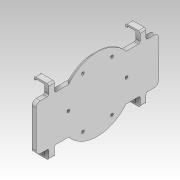
# Autodesk Inventor part: PhoneHOldER
Saved by Autodesk Inventor 2020 (Build 240168000, 168)
## iProperties
Created: 2022-08-28
Part Number: PhoneHOldER
Material: Generic
Document SubType Name: Modeling
Designer: DDeGo
Density: 1 g/cm^3
Appearance: Default
Author: DDeGo
Autodesk Inventor part; units mm, degrees
ref_plane "YZ Plane" through (0, 0, 0) normal (1, 0, 0) x (0, 1, 0)
ref_plane "XZ Plane" through (0, 0, 0) normal (0, 1, 0) x (-1, 0, 0)
sketch "Sketch1" plane through (0, 0, 0) normal (0, 0, 1) x (1, 0, 0)
  line L0 (0, 0) -> (0, 44)
  line L1 (-5, 0) -> (0, 0)
  line L2 (0, 44) -> (-1, 44)
  line L3 (-1, 44) -> (-5, 40)
  line L4 (-5, 40) -> (-5, 0)
  dimension "d0" = 44
  dimension "d3" = 1
  dimension "d19" = 5
  dimension "d20" = 45
  constraints: 10 end point, 2 horizontal, 1 perpendicular, 1 vertical
  measures "d0" distance of L0.start L0.end
  measures "d3" distance of L0.end L2.end
  measures "d19" distance between parallel lines of L0 L4
  measures "d20" angle of L0 L3
revolve "Revolution1" add sketch "Sketch1" angle 360 about axis through (-5, 0, 0) along (1, 0, 0)
sketch "Sketch2" plane through (0, 0, 0) normal (1, 0, 0) x (0, 0, -1)
  line L0 (0, 0) -> (35, 0) construction
  circle A0 centre (35, 0) radius 1.65
  dimension "d7" = 3.3
  dimension "d8" = 35
  constraints: 2 end point, 1 centre point, 1 coincident, 1 horizontal
  measures "d7" diameter of A0
  measures "d8" distance of L0.start L0.end
extrude "Extrusion1" cut sketch "Sketch2" against normal through all
ref_plane "Work Plane1" through (-2, 0, 0) normal (1, 0, 0) x (0, 0, -1)
sketch "Sketch3" plane through (-2, 0, 0) normal (1, 0, 0) x (0, 0, -1)
  circle A0 centre (35, 0) radius 3
  circle A1 centre (35, 0) radius 1.65 projected
  point P0 (0, 0)
  dimension "d12" = 6
  constraints: 1 centre point, 1 concentric
  measures "d12" diameter of A0
extrude "Extrusion2" cut sketch "Sketch3" against normal through all contours A0 | A1
pattern_circular "Circular Pattern1" count 6 over 360 about axis through (-0.5, 0, 0) along (1, 0, 0) of "Extrusion2", "Extrusion1"
sketch "Sketch4" plane through (-5, 0, 0) normal (-1, 0, 0) x (0, 0, 1)
  line L0 (73.5, 27.5) -> (-73.5, 27.5)
  line L1 (-73.5, 27.5) -> (-73.5, -27.5)
  line L2 (-73.5, -27.5) -> (73.5, -27.5)
  line L3 (73.5, -27.5) -> (73.5, 27.5)
  line L4 (73.5, 27.5) -> (-73.5, -27.5) construction
  line L5 (-73.5, 27.5) -> (73.5, -27.5) construction
  line L6 (58.5, -27.5) -> (51.5, -27.5)
  line L7 (51.5, -27.5) -> (51.5, -37.5)
  line L8 (51.5, -37.5) -> (58.5, -37.5)
  line L9 (58.5, -37.5) -> (58.5, -27.5)
  line L10 (-51.5, -27.5) -> (-58.5, -27.5)
  line L11 (-58.5, -27.5) -> (-58.5, -37.5)
  line L12 (-58.5, -37.5) -> (-51.5, -37.5)
  line L13 (-51.5, -37.5) -> (-51.5, -27.5)
  line L14 (-51.5, 27.5) -> (-58.5, 27.5)
  line L15 (-58.5, 27.5) -> (-58.5, 37.5)
  line L16 (-58.5, 37.5) -> (-51.5, 37.5)
  line L17 (-51.5, 37.5) -> (-51.5, 27.5)
  line L18 (58.5, 27.5) -> (51.5, 27.5)
  line L19 (51.5, 27.5) -> (51.5, 37.5)
  line L20 (51.5, 37.5) -> (58.5, 37.5)
  line L21 (58.5, 37.5) -> (58.5, 27.5)
  circle A0 centre (0, 0) radius 40 projected
  point P0 (-29.0474, -27.5)
  point P1 (-29.0474, 27.5)
  point P2 (29.0474, 27.5)
  point P3 (29.0474, -27.5)
  dimension "d21" = 147
  dimension "d22" = 55
  dimension "d23" = 15
  dimension "d24" = 7
  dimension "d26" = 15
  dimension "d29" = 75
  constraints: 44 end point, 10 parallel, 10 point on line, 5 horizontal, 5 perpendicular, 2 collinear, 2 midpoint
  measures "d21" distance of L1.end L2.end
  measures "d22" distance of L0.end L1.end
  measures "d23" distance between parallel lines of L3 L9
  measures "d24" distance of L7.end L8.end
  measures "d26" distance between parallel lines of L1 L11
  measures "d29" distance between parallel lines of L12 L16
extrude "Extrusion3" add sketch "Sketch4" against normal up to surface (5 mm away) contours L3 L2 A0 L0 | L0 L19 L20 L21 | L9 L8 L7 L2 | A0 L2 L1 L0 | L0 L15 L16 L17 | L13 L12 L11 L2
sketch "Sketch5" plane through (-5, 27.5, -58.5) normal (0, 0, -1) x (-1, 0, 0)
  line L0 (-5, -65) -> (10.6, -65)
  line L1 (12.6, -65) -> (12.6, -67)
  line L2 (12.6, -67) -> (-5, -67)
  line L3 (-5, -67) -> (-5, -65)
  line L4 (-5, 10) -> (10.6, 10)
  line L5 (12.6, 10) -> (12.6, 12)
  line L6 (12.6, 12) -> (-5, 12)
  line L7 (-5, 12) -> (-5, 10)
  line L8 (10.6, 10) -> (10.6, 8.5)
  line L9 (10.6, 8.5) -> (12.6, 8.5)
  line L10 (12.6, 8.5) -> (12.6, 10)
  line L11 (10.6, -65) -> (10.6, -63.5)
  line L12 (10.6, -63.5) -> (12.6, -63.5)
  line L13 (12.6, -63.5) -> (12.6, -65)
  line L14 (0, 10) -> (0, 0) projected
  point P0 (-5, -27.5)
  dimension "d30" = 2
  dimension "d31" = 10.6
  dimension "d32" = 2
  dimension "d33" = 1.5
  constraints: 28 end point, 6 parallel, 6 perpendicular, 3 equal length, 3 point on line, 2 horizontal
  measures "d30" distance between parallel lines of L4 L6
  measures "d31" distance between parallel lines of L14 L8
  measures "d32" distance of L8.end L9.end
  measures "d33" distance of L4.end L8.end
extrude "Extrusion4" add sketch "Sketch5" against normal up to surface (7 mm away)
sketch "Sketch6" plane through (-5, -37.5, 51.5) normal (0, 0, -1) x (-1, 0, 0)
  line L0 (-5, 77) -> (-5, 65) projected
  line L1 (0, 65) -> (-5, 65) projected
  line L2 (0, 75) -> (0, 65) projected
  line L3 (0, 75) -> (10.6, 75) projected
  line L4 (10.6, 75) -> (10.6, 73.5) projected
  line L5 (10.6, 73.5) -> (12.6, 73.5) projected
  line L6 (12.6, 73.5) -> (12.6, 77) projected
  line L7 (12.6, 77) -> (-5, 77) projected
  line L8 (-5, 10) -> (-5, -2) projected
  line L9 (-5, -2) -> (12.6, -2) projected
  line L10 (12.6, -2) -> (12.6, 1.5) projected
  line L11 (12.6, 1.5) -> (10.6, 1.5) projected
  line L12 (10.6, 1.5) -> (10.6, 0) projected
  line L13 (10.6, 0) -> (0, 0) projected
  line L14 (0, 10) -> (0, 0) projected
  line L15 (0, 10) -> (-5, 10) projected
  point P0 (-5, 37.5)
extrude "Extrusion5" add sketch "Sketch6" against normal up to surface (7 mm away)
fillet "Fillet1" radius 5 4 edges at (-2.5, -27.5, -73.5) (-2.5, 27.5, -73.5) (-2.5, -27.5, 73.5) (-2.5, 27.5, 73.5)
fillet "Fillet2" radius 2 4 edges at (-17.6, 39.5, 55) (-17.6, 39.5, -55) (-17.6, -39.5, 55) (-17.6, -39.5, -55)
fillet "Fillet3" radius 2 8 edges at (-2.5, 27.5, -58.5) (-2.5, 27.5, 51.5) (-2.5, -27.5, 51.5) (-2.5, -27.5, -58.5) (-2.5, -27.5, -51.5) (-2.5, -27.5, 58.5) (-2.5, 27.5, 58.5) (-2.5, 27.5, -51.5)
body "Solid1"
